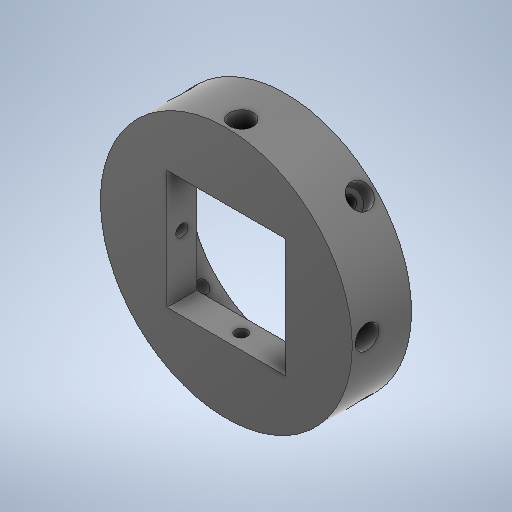
# Autodesk Inventor part: connecting_part
Saved by Autodesk Inventor 2026.2 (Build 302298010, 298A)
## iProperties
Created: 2026-04-13
Part Number: connecting_part
Material: ABS Plastic
Document SubType Name: Modeling
Designer: chris
Density: 1.06 g/cm^3
Appearance: Smooth - White
Author: chris
Autodesk Inventor part; units mm, degrees
ref_plane "YZ Plane" through (0, 0, 0) normal (1, 0, 0) x (0, 1, 0)
sketch "Sketch1" plane through (0, 0, 0) normal (0, 0, 1) x (1, 0, 0)
  circle A0 centre (0, 0) radius 42.5
  dimension "d0" = 85
  constraints: 1 centre point, 1 coincident
  measures "d0" diameter of A0
extrude "Extrusion1" add sketch "Sketch1" along normal blind 10
sketch "Sketch4" plane through (0, 0, 0) normal (0, 0, -1) x (-1, 0, 0)
  circle A0 centre (0, 0) radius 32.7
  dimension "d11" = 65.4
  constraints: 1 centre point, 1 coincident
  measures "d11" diameter of A0
extrude "Extrusion4" cut sketch "Sketch4" against normal blind 10
sketch "Sketch5" plane through (0, 0, 10) normal (0, 0, 1) x (1, 0, 0)
  circle A0 centre (0, 0) radius 42.5
  line L0 (-20.05, -20.05) -> (20.05, -20.05)
  line L1 (20.05, -20.05) -> (20.05, 20.05)
  line L2 (20.05, 20.05) -> (-20.05, 20.05)
  line L3 (-20.05, 20.05) -> (-20.05, -20.05)
  line L4 (-20.05, -20.05) -> (20.05, 20.05) construction
  line L5 (20.05, -20.05) -> (-20.05, 20.05) construction
  dimension "d14" = 85
  dimension "d15" = 40.1
  dimension "d16" = 40.1
  constraints: 12 end point, 2 midpoint, 2 parallel, 1 centre point, 1 coincident, 1 horizontal, 1 perpendicular
  measures "d14" diameter of A0
  measures "d15" distance of L2.end L1.end
  measures "d16" distance of L1.end L0.end
extrude "Extrusion5" add sketch "Sketch5" along normal blind 10
sketch "Sketch6" plane through (20.05, -19.5448, 10) normal (-1, 0, 0) x (0, 0, 1)
  circle A0 centre (5, 19.5448) radius 2.05
  line L0 (-10, -22.9552) -> (-10, 62.0448) projected
  point P0 (-10, 19.5448)
  dimension "d19" = 4.1
  dimension "d20" = 15
  constraints: 1 centre point
  measures "d19" diameter of A0
  measures "d20" distance from line of L0 A0.centre
extrude "Extrusion6" cut sketch "Sketch6" along normal through all both and the other way through all
ref_plane "Work Plane1" through (42.5, -19.5448, 10) normal (-1, 0, 0) x (0, 0, 1)
sketch "Sketch8" plane through (-19.5448, 20.05, 10) normal (0, -1, 0) x (1, 0, 0)
  circle A0 centre (19.5448, 5) radius 2.05
  line L0 (62.0448, -10) -> (-22.9552, -10) projected
  point P0 (19.5448, -10)
  dimension "d27" = 4.1
  dimension "d28" = 15
  constraints: 1 centre point
  measures "d27" diameter of A0
  measures "d28" distance from line of L0 A0.centre
extrude "Extrusion8" cut sketch "Sketch8" along normal through all both and the other way through all
ref_plane "Work Plane2" through (-19.5448, 42.5, 10) normal (0, -1, 0) x (1, 0, 0)
ref_plane "Work Plane3" through (-20.05, 20.05, 10) normal (0.7071068, 0.7071068, 0) x (0, 0, 1)
ref_plane "Work Plane4" through (-20.05, -20.05, 10) normal (-0.7071068, 0.7071068, 0) x (0, 0, 1)
ref_plane "Work Plane5" through (10.002, 50.102, 10) normal (0.7071068, 0.7071068, 0) x (0, 0, 1)
ref_plane "Work Plane6" through (-50.102, 10.002, 10) normal (-0.7071068, 0.7071068, 0) x (0, 0, 1)
sketch "Sketch10" plane through (10.002, 50.102, 10) normal (0.7071068, 0.7071068, 0) x (0, 0, 1)
  circle A0 centre (-5, 28.355) radius 2.05
  line L0 (-10, -14.145) -> (-10, 70.855) projected
  point P0 (-10, 28.355)
  dimension "d37" = 4.1
  dimension "d38" = 5
  constraints: 1 centre point
  measures "d37" diameter of A0
  measures "d38" distance from line of L0 A0.centre
extrude "Extrusion10" cut sketch "Sketch10" along normal through all both and the other way through all
sketch "Sketch12" plane through (-50.102, 10.002, 10) normal (-0.7071068, 0.7071068, 0) x (0, 0, 1)
  circle A0 centre (-5, 28.355) radius 2.05
  line L0 (-10, -14.145) -> (-10, 70.855) projected
  point P0 (-10, 28.355)
  dimension "d45" = 4.1
  dimension "d46" = 5
  constraints: 1 centre point
  measures "d45" diameter of A0
  measures "d46" distance from line of L0 A0.centre
extrude "Extrusion12" cut sketch "Sketch12" along normal through all both and the other way through all
sketch "Sketch14" plane through (42.5, -19.5448, 10) normal (-1, 0, 0) x (0, 0, 1)
  spline S0 degree 7 poles (7.05, 19.5448) (7.05, 19.8283) (7.0043, 20.1037) (6.9175, 20.3625) (6.7959, 20.5979) (6.6474, 20.8047) (6.4809, 20.9802) (6.1401, 21.2621) (5.9621, 21.3749) (5.7763, 21.4636) (5.5854, 21.5294) (5.3914, 21.573) (5.1957, 21.5948) (4.8043, 21.5948) (4.6086, 21.5729) (4.4146, 21.5294) (4.2237, 21.4636) (4.0379, 21.3749) (3.8599, 21.2621) (3.5524, 21.0078) (3.4183, 20.8722) (3.2949, 20.7173) (3.1861, 20.5438) (3.0958, 20.353) (3.0279, 20.1471) (2.9421, 19.697) (2.9286, 19.457) (2.9483, 19.2162) (3.0008, 18.9826) (3.0823, 18.7639) (3.1866, 18.5659) (3.4175, 18.2262) (3.5453, 18.0791) (3.6843, 17.9508) (3.8319, 17.841) (3.9857, 17.749) (4.144, 17.6741) (4.5422, 17.5308) (4.7857, 17.4813) (5.0323, 17.466) (5.2791, 17.4842) (5.5231, 17.5364) (5.761, 17.6238) (6.2222, 17.8773) (6.4534, 18.0509) (6.666, 18.2725) (6.8454, 18.5404) (6.9777, 18.8487) (7.05, 19.1883) (7.05, 19.5448) knots 0 0 0 0 0 0 0 0 0.127229 0.127229 0.127229 0.127229 0.127229 0.127229 0.248911 0.248911 0.248911 0.248911 0.248911 0.248911 0.370599 0.370599 0.370599 0.370599 0.370599 0.370599 0.47346 0.47346 0.47346 0.47346 0.47346 0.47346 0.582782 0.582782 0.582782 0.582782 0.582782 0.582782 0.687597 0.687597 0.687597 0.687597 0.687597 0.687597 0.841066 0.841066 0.841066 0.841066 0.841066 0.841066 1 1 1 1 1 1 1 1 projected
  circle A0 centre (5, 19.5448) radius 4
  point P0 (-10, 19.5448)
  dimension "d53" = 8
  constraints: 1 centre point, 1 other
  measures "d53" diameter of A0
extrude "Extrusion14" cut sketch "Sketch14" along normal blind 15
mirror "Mirror5" about plane through (0, 0, 0) normal (1, 0, 0) of "Extrusion14"
sketch "Sketch15" plane through (-19.5448, 42.5, 10) normal (0, -1, 0) x (1, 0, 0)
  spline S0 degree 8 poles (21.5948, 5) (21.5948, 5.2138) (21.5693, 5.4275) (21.5184, 5.6393) (21.4414, 5.8474) (21.3375, 6.0492) (21.2054, 6.2417) (21.0437, 6.4205) (20.6864, 6.7161) (20.4933, 6.8427) (20.2747, 6.9488) (20.0361, 7.0262) (19.7846, 7.0697) (19.5284, 7.0767) (19.276, 7.0475) (18.7866, 6.9218) (18.5585, 6.8254) (18.3532, 6.703) (18.1721, 6.56) (18.0155, 6.4015) (17.8835, 6.2316) (17.7752, 6.0543) (17.5844, 5.6486) (17.5126, 5.4158) (17.4729, 5.1781) (17.4644, 4.9383) (17.4869, 4.6988) (17.5409, 4.4623) (17.6276, 4.232) (17.8384, 3.8485) (17.9483, 3.689) (18.0789, 3.5369) (18.2303, 3.3955) (18.4026, 3.2683) (18.5951, 3.1593) (18.8066, 3.073) (19.2576, 2.9572) (19.4908, 2.9278) (19.7283, 2.9292) (19.963, 2.9622) (20.188, 3.025) (20.397, 3.1137) (20.5853, 3.2221) (20.9687, 3.5006) (21.153, 3.685) (21.3032, 3.8865) (21.4211, 4.0995) (21.5083, 4.3201) (21.5659, 4.5452) (21.5948, 4.7725) (21.5948, 5) knots 0 0 0 0 0 0 0 0 0 0.153736 0.153736 0.153736 0.153736 0.153736 0.153736 0.153736 0.285695 0.285695 0.285695 0.285695 0.285695 0.285695 0.285695 0.421636 0.421636 0.421636 0.421636 0.421636 0.421636 0.421636 0.589625 0.589625 0.589625 0.589625 0.589625 0.589625 0.589625 0.714964 0.714964 0.714964 0.714964 0.714964 0.714964 0.714964 0.837183 0.837183 0.837183 0.837183 0.837183 0.837183 0.837183 1 1 1 1 1 1 1 1 1 projected
  circle A0 centre (19.5448, 5) radius 4
  point P0 (19.5448, -10)
  dimension "d56" = 8
  constraints: 1 centre point, 1 other
  measures "d56" diameter of A0
extrude "Extrusion15" cut sketch "Sketch15" along normal blind 15
mirror "Mirror6" about plane through (0, 0, 0) normal (0, 1, 0) of "Extrusion15"
sketch "Sketch16" plane through (-50.102, 10.002, 10) normal (-0.7071068, 0.7071068, 0) x (0, 0, 1)
  spline S0 degree 8 poles (-2.95, 28.355) (-2.95, 28.6031) (-2.9843, 28.8451) (-3.05, 29.0757) (-3.1433, 29.2904) (-3.2598, 29.4857) (-3.3942, 29.6588) (-3.5408, 29.8084) (-3.8391, 30.0551) (-3.9934, 30.1569) (-4.154, 30.2406) (-4.3191, 30.3067) (-4.4874, 30.3559) (-4.6575, 30.3886) (-4.8287, 30.405) (-5.2138, 30.405) (-5.4275, 30.3795) (-5.6393, 30.3286) (-5.8474, 30.2517) (-6.0492, 30.1478) (-6.2417, 30.0157) (-6.4205, 29.854) (-6.7161, 29.4967) (-6.8427, 29.3035) (-6.9488, 29.0849) (-7.0262, 28.8463) (-7.0697, 28.5948) (-7.0767, 28.3386) (-7.0475, 28.0862) (-6.9456, 27.6892) (-6.8915, 27.5369) (-6.8239, 27.3896) (-6.7431, 27.2488) (-6.6501, 27.1158) (-6.5456, 26.9918) (-6.4308, 26.8781) (-6.1703, 26.6625) (-6.0226, 26.5631) (-5.8654, 26.4785) (-5.7004, 26.4096) (-5.5293, 26.3574) (-5.3542, 26.3225) (-5.1771, 26.305) (-4.8287, 26.305) (-4.6575, 26.3213) (-4.4874, 26.354) (-4.3191, 26.4032) (-4.154, 26.4694) (-3.9934, 26.553) (-3.8391, 26.6548) (-3.5409, 26.9015) (-3.3943, 27.0511) (-3.2597, 27.2243) (-3.1432, 27.4196) (-3.0499, 27.6344) (-2.9843, 27.8651) (-2.95, 28.107) (-2.95, 28.355) knots 0 0 0 0 0 0 0 0 0 0.142663 0.142663 0.142663 0.142663 0.142663 0.142663 0.142663 0.279107 0.279107 0.279107 0.279107 0.279107 0.279107 0.279107 0.449413 0.449413 0.449413 0.449413 0.449413 0.449413 0.449413 0.595594 0.595594 0.595594 0.595594 0.595594 0.595594 0.595594 0.690173 0.690173 0.690173 0.690173 0.690173 0.690173 0.690173 0.794213 0.794213 0.794213 0.794213 0.794213 0.794213 0.794213 0.894835 0.894835 0.894835 0.894835 0.894835 0.894835 0.894835 1 1 1 1 1 1 1 1 1 projected
  circle A0 centre (-5, 28.355) radius 4
  point P0 (-10, 28.355)
  dimension "d59" = 8
  constraints: 1 centre point, 1 other
  measures "d59" diameter of A0
extrude "Extrusion16" cut sketch "Sketch16" against normal blind 5
mirror "Mirror7" about plane through (-20.05, -20.05, 10) normal (-0.7071068, 0.7071068, 0) of "Extrusion16"
sketch "Sketch17" plane through (10.002, 50.102, 10) normal (0.7071068, 0.7071068, 0) x (0, 0, 1)
  spline S0 degree 8 poles (-2.95, 28.355) (-2.95, 28.6031) (-2.9843, 28.8451) (-3.05, 29.0757) (-3.1433, 29.2904) (-3.2598, 29.4857) (-3.3942, 29.6588) (-3.5408, 29.8084) (-3.8391, 30.0551) (-3.9934, 30.1569) (-4.154, 30.2406) (-4.3191, 30.3067) (-4.4874, 30.3559) (-4.6575, 30.3886) (-4.8287, 30.405) (-5.2138, 30.405) (-5.4275, 30.3795) (-5.6393, 30.3286) (-5.8474, 30.2517) (-6.0492, 30.1478) (-6.2417, 30.0157) (-6.4205, 29.854) (-6.7161, 29.4967) (-6.8427, 29.3035) (-6.9488, 29.0849) (-7.0262, 28.8463) (-7.0697, 28.5948) (-7.0767, 28.3386) (-7.0475, 28.0862) (-6.9456, 27.6892) (-6.8915, 27.5369) (-6.8239, 27.3896) (-6.7431, 27.2488) (-6.6501, 27.1158) (-6.5456, 26.9918) (-6.4308, 26.8781) (-6.1703, 26.6625) (-6.0226, 26.5631) (-5.8654, 26.4785) (-5.7004, 26.4096) (-5.5293, 26.3574) (-5.3542, 26.3225) (-5.1771, 26.305) (-4.8287, 26.305) (-4.6575, 26.3213) (-4.4874, 26.354) (-4.3191, 26.4032) (-4.154, 26.4694) (-3.9934, 26.553) (-3.8391, 26.6548) (-3.5409, 26.9015) (-3.3943, 27.0511) (-3.2597, 27.2243) (-3.1432, 27.4196) (-3.0499, 27.6344) (-2.9843, 27.8651) (-2.95, 28.107) (-2.95, 28.355) knots 0 0 0 0 0 0 0 0 0 0.142663 0.142663 0.142663 0.142663 0.142663 0.142663 0.142663 0.279107 0.279107 0.279107 0.279107 0.279107 0.279107 0.279107 0.449413 0.449413 0.449413 0.449413 0.449413 0.449413 0.449413 0.595594 0.595594 0.595594 0.595594 0.595594 0.595594 0.595594 0.690173 0.690173 0.690173 0.690173 0.690173 0.690173 0.690173 0.794213 0.794213 0.794213 0.794213 0.794213 0.794213 0.794213 0.894835 0.894835 0.894835 0.894835 0.894835 0.894835 0.894835 1 1 1 1 1 1 1 1 1 projected
  circle A0 centre (-5, 28.355) radius 4
  point P0 (-10, 28.355)
  dimension "d62" = 8
  constraints: 1 centre point, 1 other
  measures "d62" diameter of A0
extrude "Extrusion17" cut sketch "Sketch17" against normal blind 5
mirror "Mirror8" about plane through (-20.05, 20.05, 10) normal (0.7071068, 0.7071068, 0) of "Extrusion17"
body "Solid1"
